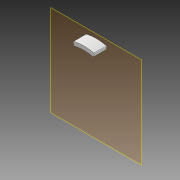
# Autodesk Inventor part: Стойка
Saved by Autodesk Inventor 2022 (Build 260153000, 153)
## iProperties
Created: 2025-01-11
Part Number: Стойка
Material: Типовые
Document SubType Name: Modeling
Designer: Ivan
Density: 1 g/cm^3
Appearance: По умолчанию
Author: Ivan
Autodesk Inventor part; units mm, degrees
ref_plane "YZ Plane" through (0, 0, 0) normal (1, 0, 0) x (0, 1, 0)
ref_plane "XZ Plane" through (0, 0, 0) normal (0, 1, 0) x (-1, 0, 0)
ref_plane "РабПлоскость1" through (0, 0, -57.3048) normal (0, 0, 1) x (-1, 0, 0)
sketch "Эскиз1" plane through (0, 0, -57.3048) normal (0, 0, 1) x (-1, 0, 0)
  circle A0 centre (0, 0) radius 132.5 projected
  line L0 (31.1877, -116.3941) -> (34.2935, -127.9852) projected
  arc A1 (-31.1877, -116.3941) -> (31.1877, -116.3941) centre (0, 0) ccw projected
  line L1 (-34.2935, -127.9852) -> (-31.1877, -116.3941) projected
  point P0 (0, 0)
ref_plane "РабПлоскость2" through (-132.2012, -132.5, -3) normal (0, 0, -1) x (0, 1, 0)
extrude "Выдавливание1" add sketch "Эскиз1" along normal blind 40 contours L1 A1 L0 A0 picked at (24.6238, -125.9568)
fillet "Сопряжение1" radius 2 4 edges at (34.2935, 127.9852, -37.3048) (31.1877, 116.3941, -37.3048) (-31.1877, 116.3941, -37.3048) (-34.2935, 127.9852, -37.3048)
